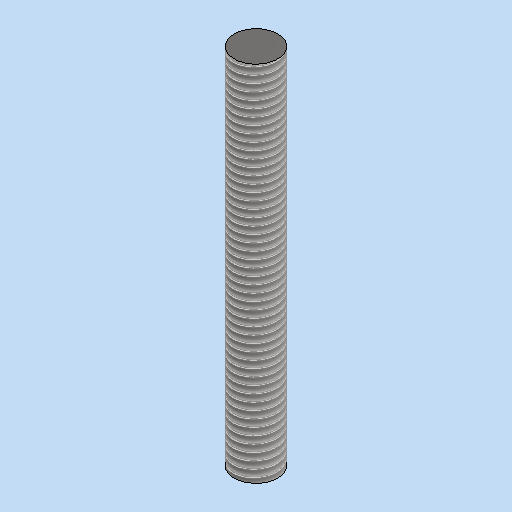
# Autodesk Inventor part: boron target m3 pin
Saved by Autodesk Inventor 2025 (Build 290162000, 162)
## iProperties
Created: 2020-09-07
Part Number: boron target m3 pin
Material: Stainless Steel
Document SubType Name: Modeling
Designer: mkse
Density: 8 g/cm^3
Appearance: Semi-Polished
Author: mkse
Autodesk Inventor part; units mm, degrees
ref_plane "YZ Plane" through (0, 0, 0) normal (1, 0, 0) x (0, 1, 0)
ref_plane "XZ Plane" through (0, 0, 0) normal (0, 1, 0) x (-1, 0, 0)
ref_plane "XY Plane" through (0, 0, 0) normal (0, 0, 1) x (1, 0, 0)
sketch "sketch1" plane through (0, 0, 0) normal (0, 1, 0) x (-1, 0, 0)
  circle A0 centre (0, 0) radius 1.5
  dimension "d0" = 3
  constraints: 1 centre point, 1 coincident
  measures "d0" diameter of A0
extrude "押し出し1" add sketch "sketch1" along normal blind 10 and the other way blind 15
thread "Thread1" size "M3x0.5" class "6g" standard "ANSI Metric M Profile" full length
